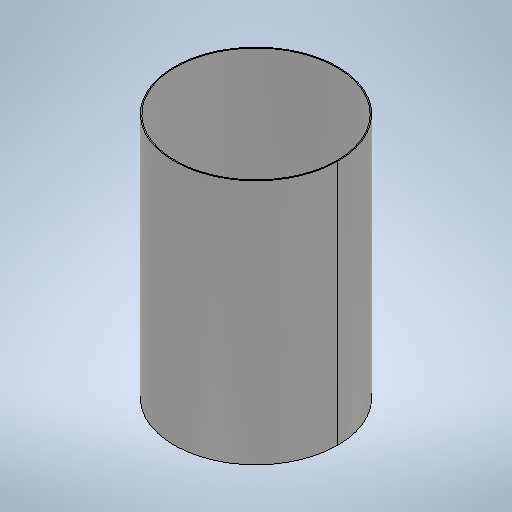
# Autodesk Inventor part: TKS 3102 TOP DS main tube
Saved by Autodesk Inventor 2025.3 (Build 293356030, 356C)
## iProperties
Created: 2025-02-19
Part Number: TKS 3102 TOP DS main tube
Material: Stainless Steel
Document SubType Name: Sheet Metal
Designer: user
Density: 8 g/cm^3
Appearance: Semi-Polished
Flat Pattern Width: 23 cm
Flat Pattern Length: 47.7013 cm
Flat Pattern Area: 1097.13 cm^2
Sheet Metal Rule: Default_mm
Sheet Metal Width: 230,000 mm
Sheet Metal Length: 477,013 mm
Sheet Metal Area: 109712,887 mm^2
Author: admin
Autodesk Inventor part; units mm, degrees
ref_plane "YZ Plane" through (0, 0, 0) normal (1, 0, 0) x (0, 1, 0)
ref_plane "XZ Plane" through (0, 0, 0) normal (0, 1, 0) x (-1, 0, 0)
ref_plane "XY Plane" through (0, 0, 0) normal (0, 0, 1) x (1, 0, 0)
sketch "Sketch2" plane through (0, 0, 0) normal (0, 1, 0) x (-1, 0, 0)
  line L0 (-75.5, 230) -> (-76.5, 230)
  line L1 (-76.5, 230) -> (-76.5, 0)
  line L2 (-76.5, 0) -> (-75.5, 0)
  line L3 (-75.5, 0) -> (-75.5, 230)
  line L4 (0, 0) -> (0, 230)
  point P0 (-76, 0)
  point P1 (-76, 230)
  dimension "d4" = 230
  dimension "d5" = 1
  dimension "d6" = 153
  constraints: 10 end point, 2 horizontal alignment, 2 midpoint, 2 parallel, 1 horizontal, 1 perpendicular, 1 vertical
  measures "d4" distance of L4.start L4.end
  measures "d5" distance of L0.start L0.end
  measures "d6" diameter of L1 L4
revolve "Revolution1" add sketch "Sketch2" angle 359.9 about axis through (0, 0, 0) along (0, 0, 1)
equation "\"BendRadius\" = Thickness"
equation "\"BendReliefWidth\" = Thickness"
equation "\"BendReliefDepth\" = 0.5 * Thickness"
equation "\"CornerReliefSize\" = 4 * Thickness"
equation "\"MinimumRemnant\" = 2 * Thickness"
equation "\"TransitionRadius\" = BendRadius"
equation "\"JacobiRadiusSize\" = BendRadius"
equation "\"GapSize\" = Thickness"
equation "\"Thickness\" = 1"
body "Solid2"
